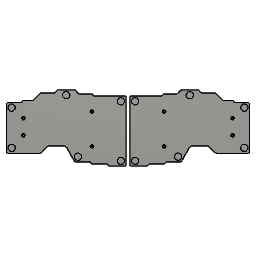
mriya-cnc-bottom-plate-v.1.00 (Autodesk Fusion 360 design; units mm, degrees)
Autodesk Fusion 360 part; units mm, degrees
sketch "mriya-bottom-plate" plane through (0, 0, 0) normal (0, 0, 1) x (1, 0, 0)
  line L0 (-96.0213, 15.6719) -> (-89.7787, 21.9145)
  line L1 (-21.4858, 1.079) -> (-22.6142, 2.2074)
  line L2 (-133.1, 14.7932) -> (-98.1426, 14.7932)
  line L3 (-39.0716, 2.7932) -> (-24.0284, 2.7932)
  line L4 (-3.6, 0.4932) -> (-20.0716, 0.4932)
  line L5 (-59.4741, 6.1094) -> (-67.7517, 20.7608)
  line L6 (-40.4858, 3.379) -> (-41.6142, 4.5074)
  line L7 (-117.6142, 71.579) -> (-116.4858, 72.7074)
  line L8 (-96.0716, 81.2932) -> (-82.2284, 81.2932)
  line L9 (-133.1, 70.9932) -> (-119.0284, 70.9932)
  line L10 (-87.6574, 22.7932) -> (-71.2344, 22.7932)
  line L11 (-43.0284, 5.0932) -> (-57.7328, 5.0932)
  line L12 (-104.3142, 73.879) -> (-97.4858, 80.7074)
  line L13 (-77.0716, 84.7932) -> (-59.7284, 84.7932)
  line L14 (-53.5716, 80.2932) -> (-40.7284, 80.2932)
  line L15 (-105.7284, 73.2932) -> (-115.0716, 73.2932)
  line L16 (-78.4858, 84.2074) -> (-80.8142, 81.879)
  line L17 (-58.3142, 84.2074) -> (-54.9858, 80.879)
  line L18 (-134.6, 69.4932) -> (-134.6, 16.2932)
  line L19 (-38.1858, 78.579) -> (-39.3142, 79.7074)
  circle A0 centre (-115.9, 53.5432) radius 1
  circle A1 centre (-115.9, 34.5432) radius 1
  circle A2 centre (-39.9, 22.5432) radius 1
  circle A3 centre (-39.9, 60.5432) radius 1
  arc A4 (-38.1858, 78.579) -> (-36.7716, 77.9932) centre (-36.7716, 79.9932) ccw
  arc A5 (-39.3142, 79.7074) -> (-40.7284, 80.2932) centre (-40.7284, 78.2932) ccw
  arc A6 (-54.9858, 80.879) -> (-53.5716, 80.2932) centre (-53.5716, 82.2931) ccw
  arc A7 (-58.3142, 84.2074) -> (-59.7284, 84.7932) centre (-59.7284, 82.7932) ccw
  arc A8 (-77.0716, 84.7932) -> (-78.4858, 84.2074) centre (-77.0716, 82.7933) ccw
  arc A9 (-82.2284, 81.2932) -> (-80.8142, 81.879) centre (-82.2284, 83.2932) ccw
  arc A10 (-96.0716, 81.2932) -> (-97.4858, 80.7074) centre (-96.0716, 79.2933) ccw
  arc A11 (-105.7284, 73.2932) -> (-104.3142, 73.879) centre (-105.7284, 75.2932) ccw
  arc A12 (-115.0716, 73.2932) -> (-116.4858, 72.7074) centre (-115.0716, 71.2933) ccw
  arc A13 (-119.0284, 70.9932) -> (-117.6142, 71.579) centre (-119.0284, 72.9932) ccw
  arc A14 (-133.1, 70.9932) -> (-134.6, 69.4932) centre (-133.1, 69.4932) ccw
  arc A15 (-134.6, 16.2932) -> (-133.1, 14.7932) centre (-133.1, 16.2932) ccw
  arc A16 (-98.1426, 14.7932) -> (-96.0213, 15.6719) centre (-98.1426, 17.7931) ccw
  arc A17 (-87.6574, 22.7932) -> (-89.7787, 21.9145) centre (-87.6573, 19.7931) ccw
  arc A18 (-67.7517, 20.7608) -> (-71.2344, 22.7932) centre (-71.2344, 18.793) ccw
  arc A19 (-59.4741, 6.1094) -> (-57.7328, 5.0932) centre (-57.7328, 7.0932) ccw
  arc A20 (-41.6142, 4.5074) -> (-43.0284, 5.0932) centre (-43.0284, 3.0933) ccw
  arc A21 (-40.4858, 3.379) -> (-39.0716, 2.7932) centre (-39.0716, 4.7932) ccw
  arc A22 (-22.6142, 2.2074) -> (-24.0284, 2.7932) centre (-24.0284, 0.7933) ccw
  arc A23 (-21.4858, 1.079) -> (-20.0716, 0.4932) centre (-20.0716, 2.4932) ccw
  arc A24 (-3.6, 0.4932) -> (-2.1, 1.9932) centre (-3.6, 1.9932) ccw
  line L20 (-2.1, 1.9932) -> (-2.1, 76.4932)
  line L21 (-36.7716, 77.9932) -> (-3.6, 77.9932)
  arc A25 (-2.1, 76.4932) -> (-3.6, 77.9932) centre (-3.6, 76.4932) ccw
  circle A26 centre (-115.9, 53.5432) radius 2
  circle A27 centre (-115.9, 34.5432) radius 2
  circle A28 centre (-39.9, 22.5432) radius 2
  circle A29 centre (-39.9, 60.5432) radius 2
  circle A30 centre (-128.8, 20.5932) radius 4.05
  circle A31 centre (-128.8, 65.1932) radius 4.05
  circle A32 centre (-68.4, 78.9932) radius 4.05
  circle A33 centre (-7.9, 72.1932) radius 4.05
  circle A34 centre (-7.9, 6.2932) radius 4.05
  circle A35 centre (-55.5152, 10.8932) radius 4.05
  arc A36 (-54.9504, 80.9144) -> (-53.5716, 80.3432) centre (-53.5716, 82.2931) ccw
  line L22 (-53.5716, 80.3432) -> (-40.7284, 80.3432)
  arc A37 (-39.2788, 79.7428) -> (-40.7284, 80.3432) centre (-40.7284, 78.2932) ccw
  line L23 (-38.1504, 78.6144) -> (-39.2788, 79.7428)
  arc A38 (-38.1504, 78.6144) -> (-36.7716, 78.0432) centre (-36.7716, 79.9932) ccw
  line L24 (-36.7716, 78.0432) -> (-3.6, 78.0432)
  arc A39 (-2.05, 76.4932) -> (-3.6, 78.0432) centre (-3.6, 76.4932) ccw
  line L25 (-2.05, 1.9932) -> (-2.05, 76.4932)
  arc A40 (-3.6, 0.4432) -> (-2.05, 1.9932) centre (-3.6, 1.9932) ccw
  line L26 (-3.6, 0.4432) -> (-20.0716, 0.4432)
  arc A41 (-21.5212, 1.0436) -> (-20.0716, 0.4432) centre (-20.0716, 2.4932) ccw
  line L27 (-21.5212, 1.0436) -> (-22.6496, 2.172)
  arc A42 (-22.6496, 2.172) -> (-24.0284, 2.7432) centre (-24.0284, 0.7933) ccw
  line L28 (-39.0716, 2.7432) -> (-24.0284, 2.7432)
  arc A43 (-40.5212, 3.3436) -> (-39.0716, 2.7432) centre (-39.0716, 4.7932) ccw
  line L29 (-40.5212, 3.3436) -> (-41.6496, 4.472)
  arc A44 (-41.6496, 4.472) -> (-43.0284, 5.0432) centre (-43.0284, 3.0933) ccw
  line L30 (-43.0284, 5.0432) -> (-57.7328, 5.0432)
  arc A45 (-59.5176, 6.0848) -> (-57.7328, 5.0432) centre (-57.7328, 7.0932) ccw
  line L31 (-59.5176, 6.0848) -> (-67.7952, 20.7362)
  arc A46 (-67.7952, 20.7362) -> (-71.2344, 22.7432) centre (-71.2344, 18.793) ccw
  line L32 (-87.6574, 22.7432) -> (-71.2344, 22.7432)
  arc A47 (-87.6574, 22.7432) -> (-89.7433, 21.8791) centre (-87.6573, 19.7931) ccw
  line L33 (-95.9859, 15.6365) -> (-89.7433, 21.8791)
  arc A48 (-98.1426, 14.7432) -> (-95.9859, 15.6365) centre (-98.1426, 17.7931) ccw
  line L34 (-133.1, 14.7432) -> (-98.1426, 14.7432)
  arc A49 (-134.65, 16.2932) -> (-133.1, 14.7432) centre (-133.1, 16.2932) ccw
  line L35 (-134.65, 69.4932) -> (-134.65, 16.2932)
  arc A50 (-133.1, 71.0432) -> (-134.65, 69.4932) centre (-133.1, 69.4932) ccw
  line L36 (-133.1, 71.0432) -> (-119.0284, 71.0432)
  arc A51 (-119.0284, 71.0432) -> (-117.6496, 71.6144) centre (-119.0284, 72.9932) ccw
  line L37 (-117.6496, 71.6144) -> (-116.5212, 72.7428)
  arc A52 (-115.0716, 73.3432) -> (-116.5212, 72.7428) centre (-115.0716, 71.2933) ccw
  line L38 (-105.7284, 73.3432) -> (-115.0716, 73.3432)
  arc A53 (-105.7284, 73.3432) -> (-104.3496, 73.9144) centre (-105.7284, 75.2932) ccw
  line L39 (-104.3496, 73.9144) -> (-97.5212, 80.7428)
  arc A54 (-96.0716, 81.3432) -> (-97.5212, 80.7428) centre (-96.0716, 79.2933) ccw
  line L40 (-96.0716, 81.3432) -> (-82.2284, 81.3432)
  arc A55 (-82.2284, 81.3432) -> (-80.8496, 81.9144) centre (-82.2284, 83.2932) ccw
  line L41 (-78.5212, 84.2428) -> (-80.8496, 81.9144)
  arc A56 (-77.0716, 84.8432) -> (-78.5212, 84.2428) centre (-77.0716, 82.7933) ccw
  line L42 (-77.0716, 84.8432) -> (-59.7284, 84.8432)
  arc A57 (-58.2788, 84.2428) -> (-59.7284, 84.8432) centre (-59.7284, 82.7932) ccw
  line L43 (-58.2788, 84.2428) -> (-54.9504, 80.9144)
  dimension "d1" = 2
  dimension "d2" = 2
  dimension "d4" = 2
  dimension "d5" = 2
  dimension "d15" = 4
  dimension "d16" = 4
  dimension "d17" = 4
  dimension "d18" = 4
  dimension "d19" = 8.1
  dimension "d20" = 8.1
  dimension "d21" = 8.1
  dimension "d22" = 8.1
  dimension "d23" = 8.1
  dimension "d24" = 8.1
  dimension "d25" = 5.8
  dimension "d26" = 5.8
  dimension "d27" = 5.8
  dimension "d28" = 5.8
  dimension "d29" = 5.8
  dimension "d30" = 5.8
  dimension "d31" = 5.8
  dimension "d32" = 5.8
  dimension "d33" = 5.8
  dimension "d34" = 5.8
  dimension "d35" = 5.8
  dimension "d42" = -0.05
  constraint tangent L19 A4
  constraint tangent L19 A5
  constraint tangent L14 A6
  constraint tangent L17 A7
  constraint tangent L13 A8
  constraint tangent L16 A9
  constraint tangent L8 A10
  constraint tangent L12 A11
  constraint tangent L15 A12
  constraint tangent L7 A13
  constraint tangent L9 A14
  constraint tangent L18 A15
  constraint tangent L2 A16
  constraint tangent L0 A17
  constraint tangent L10 A18
  constraint tangent L5 A19
  constraint tangent L11 A20
  constraint tangent L6 A21
  constraint tangent L3 A22
  constraint tangent L1 A23
  constraint tangent L4 A24
  constraint tangent A24 L20
  constraint perpendicular L20 L21
  constraint tangent L20 A25
  constraint tangent L21 A25
  constraint concentric A0 A26
  constraint concentric A1 A27
  constraint concentric A2 A28
  constraint concentric A3 A29
  measures "d1" diameter of A0
  measures "d2" diameter of A1
  measures "d4" diameter of A2
  measures "d5" diameter of A3
  measures "d15" diameter of A26
  measures "d16" diameter of A27
  measures "d17" diameter of A28
  measures "d18" diameter of A29
  measures "d19" diameter of A30
  measures "d20" diameter of A31
  measures "d21" diameter of A32
  measures "d22" diameter of A33
  measures "d23" diameter of A34
  measures "d24" diameter of A35
  measures "d25" distance of L9 A31.centre
  measures "d26" distance of L18 A31.centre
  measures "d27" distance of L13 A32.centre
  measures "d28" distance of L21 A33.centre
  measures "d29" distance of L20 A33.centre
  measures "d30" distance of L20 A34.centre
  measures "d31" distance of L4 A34.centre
  measures "d32" distance of L11 A35.centre
  measures "d33" distance of L5 A35.centre
  measures "d34" distance of L2 A30.centre
  measures "d35" distance of L18 A30.centre
extrude "Extrude1" add sketch "mriya-bottom-plate" along normal blind 1.5 contours L0 L1 L2 L3 L4 L5 L6 L7 L8 L9 L10 L11 L12 L13 L14 L15 L16 L17 L18 L19 A4 A5 A6 A7 A8 A9 A10 A11 A12 A13 A14 A15 A16 A17 A18 A19 A20 A21 A22 A23 A24 L20 L21 A25 | A36 L22 A37 L23 A38 L24 A39 L25 A40 L26 A41 L27 A42 L28 A43 L29 A44 L30 A45 L31 A46 L32 A47 L33 A48 L34 A49 L35 A50 L36 A51 L37 A52 L38 A53 L39 A54 L40 A55 L41 A56 L42 A57 L43 makes body 1
extrude "Extrude2" add sketch "mriya-bottom-plate" along normal blind 0.7 contours A26 | A27 | A28 | A29 | A30 | A31 | A32 | A33 | A34 | A35 bodies 1
mirror "Mirror1" about plane through (0, 0, 0) normal (1, 0, 0) of bodies 1 makes body 2
named bodies: "Left", "Right"
